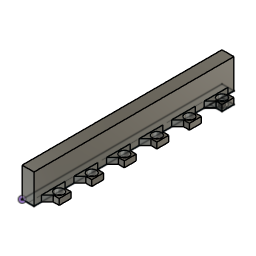
Divider v2 (Autodesk Fusion 360 design; units mm, degrees)
Autodesk Fusion 360 part; units mm, degrees
sketch "Sketch1" plane through (0, 0, 0) normal (0, 0, 1) x (1, 0, 0)
  line L0 (0, 0) -> (0, 135)
  line L1 (0, 135) -> (8, 135)
  line L2 (8, 135) -> (8, 0)
  line L3 (8, 0) -> (0, 0)
  line L4 (8, 135) -> (8, 127) construction
  line L5 (8, 127) -> (16, 127)
  line L6 (16, 127) -> (16, 119)
  line L7 (16, 119) -> (8, 119)
  line L8 (8, 119) -> (8, 127)
  line L9 (4, 135) -> (4, 0) construction
  line L10 (12, 127) -> (8, 131)
  line L11 (12, 119) -> (8, 115)
  line L12 (12, 119) -> (12, 127) construction
  circle A0 centre (12, 123) radius 3.15
  line L13 (8, 131) -> (8, 115)
  dimension "d1" = 135
  dimension "d2" = 8
  dimension "d3" = 8
  dimension "d4" = 8
  dimension "d5" = 8
  dimension "d6" = 6.3
  constraint coincident L0.start L3.end
  constraint vertical L0
  constraint perpendicular L0 L1
  constraint perpendicular L1 L2
  constraint perpendicular L0 L3
  constraint perpendicular L1 L4
  constraint horizontal L5
  constraint vertical L6
  constraint horizontal L7
  constraint vertical L8
  constraint midpoint L1 L9.start
  constraint midpoint L3 L9.end
  constraint midpoint L5 L10.start
  constraint midpoint L4 L10.end
  constraint midpoint L7 L11.start
  constraint coincident L2 L11.end
  constraint perpendicular L10 L11
  constraint midpoint L12 A0.centre
  measures "d1" distance of L0.start L0.end
  measures "d2" distance of L0.end L1.end
  measures "d3" distance of L1.end L4.end
  measures "d4" distance of L4.end L5.end
  measures "d5" distance of L4.end L7.end
  measures "d6" diameter of A0
extrude "Extrude1" add sketch "Sketch1" along normal blind 20 contours L0 L1 L2 L3 L8 L13 makes body 1
extrude "Extrude2" add sketch "Sketch1" along normal blind 4 separate body contours L2 L7 L11 L13 | L2 L5 L10 L13 | L2 L5 L6 L7 L8 L13 makes body 2
pattern_linear "R-Pattern1" count 6 spacing 22 along (0, -1, 0) of bodies 2 makes body 3 at (15.1461, 100.843, 2.6667) makes body 4 at (15.1461, 78.843, 2.6667) makes body 5 at (8.8657, 56.6864, 2.6667) makes body 6 at (8.8657, 34.6864, 2.6667) makes body 7 at (15.1461, 12.843, 2.6667)
sketch "Sketch2" plane through (0, 0, 20) normal (0, 0, 1) x (-1, 0, 0)
  line L0 (-8, 0) -> (-8, -135)
  line L1 (-8, -135) -> (0, -135)
  line L2 (0, -135) -> (0, 0)
  line L3 (0, 0) -> (-8, 0)
  line L4 (-4, 0) -> (-4, -135)
  constraint midpoint L1 L4.end
ref_plane "WorkPlane1" through (4, 67.5, 10) normal (1, 0, 0) x (0, 1, 0)
mirror "Mirror1" about plane through (4, 67.5, 10) normal (1, 0, 0) of bodies 2 3 4 5 6 7 makes body 8 at (-7.1461, 122.843, 2.6667) makes body 9 at (-7.1461, 100.843, 2.6667) makes body 10 at (-7.1461, 78.843, 2.6667) makes body 11 at (-0.8657, 56.6864, 2.6667) makes body 12 at (-0.8657, 34.6864, 2.6667) makes body 13 at (-7.1461, 12.843, 2.6667)
combine "Combine1" operation add target body 1 tool bodies 8 9 10 11 12 13 6 7 5 4 3 2
